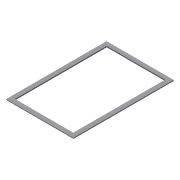
# Autodesk Inventor part: lowerGom
Saved by Autodesk Inventor 2014 (Build 180170000, 170)
## iProperties
Created: 2014-05-05
Part Number: lowerGom
Material: 一般
Document SubType Name: Modeling
Designer: motegi
Density: 1 g/cm^3
Appearance: 既定
Author: motegi
Autodesk Inventor part; units mm, degrees
ref_plane "YZ Plane" through (0, 0, 0) normal (1, 0, 0) x (0, 1, 0)
ref_plane "XZ Plane" through (0, 0, 0) normal (0, 1, 0) x (-1, 0, 0)
ref_plane "XY Plane" through (0, 0, 0) normal (0, 0, 1) x (1, 0, 0)
sketch "スケッチ1" plane through (0, 0, 0) normal (0, 0, 1) x (1, 0, 0)
  line L0 (-231, 344) -> (231, 344)
  line L1 (231, 344) -> (231, -344)
  line L2 (231, -344) -> (-231, -344)
  line L3 (-231, -344) -> (-231, 344)
  line L4 (-231, 344) -> (231, -344) construction
  line L5 (231, 344) -> (-231, -344) construction
  point P0 (0, 0)
  dimension "d0" = 462
  dimension "d1" = 688
  constraints: 12 end point, 2 midpoint, 2 parallel, 1 horizontal, 1 perpendicular
  measures "d0" distance of L1.end L2.end
  measures "d1" distance of L0.end L1.end
extrude "押し出し1" add sketch "スケッチ1" along normal blind 8.35
sketch "スケッチ2" plane through (0, 0, 8.35) normal (0, 0, 1) x (1, 0, 0)
  line L0 (-200, -314.5) -> (200, -314.5)
  line L1 (200, -314.5) -> (200, 314.5)
  line L2 (200, 314.5) -> (-200, 314.5)
  line L3 (-200, 314.5) -> (-200, -314.5)
  line L4 (-200, -314.5) -> (200, 314.5) construction
  line L5 (200, -314.5) -> (-200, 314.5) construction
  point P0 (0, 0)
  dimension "d4" = 400
  dimension "d5" = 629
  constraints: 12 end point, 2 midpoint, 2 parallel, 1 horizontal, 1 perpendicular
  measures "d4" distance of L2.end L1.end
  measures "d5" distance of L1.end L0.end
extrude "押し出し2" cut sketch "スケッチ2" against normal blind 8.35
fillet "フィレット1" radius 3 11 edges at (231, 344, 4.175) (231, 0, 8.35) (0, 344, 8.35) (0, 344, 0) (231, 0, 0) (-231, 344, 4.175) (-231, 0, 8.35) (-231, 0, 0) (-231, -344, 4.175) (0, -344, 8.35) (0, -344, 0)
